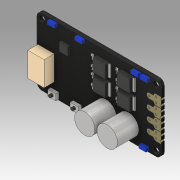
# Autodesk Inventor part: motorcontroller
Saved by Autodesk Inventor 2019.3 (Build 233278000, 278)
## iProperties
Created: 2019-05-13
Part Number: motorcontroller
Material: Generic
Document SubType Name: Modeling
Designer: Dave
Density: 1 g/cm^3
Appearance: Default
Author: Dave
Autodesk Inventor part; units mm, degrees
ref_plane "YZ Plane" through (0, 0, 0) normal (1, 0, 0) x (0, 1, 0)
ref_plane "XZ Plane" through (0, 0, 0) normal (0, 1, 0) x (-1, 0, 0)
ref_plane "XY Plane" through (0, 0, 0) normal (0, 0, 1) x (1, 0, 0)
sketch "Sketch1" plane through (0, 0, 0) normal (0, 0, 1) x (1, 0, 0)
  line L0 (2.5, 0) -> (58.5, 0)
  line L1 (61, 2.5) -> (61, 30.5)
  line L2 (58.5, 33) -> (2.5, 33)
  line L3 (0, 30.5) -> (0, 2.5)
  arc A0 (2.5, 33) -> (0, 30.5) centre (2.5, 30.5) ccw
  arc A1 (61, 30.5) -> (58.5, 33) centre (58.5, 30.5) ccw
  arc A2 (58.5, 0) -> (61, 2.5) centre (58.5, 2.5) ccw
  arc A3 (0, 2.5) -> (2.5, 0) centre (2.5, 2.5) ccw
  circle A4 centre (2.5, 30.5) radius 1.5
  circle A5 centre (2.5, 2.5) radius 1.5
  circle A6 centre (58.5, 30.5) radius 1.5
  circle A7 centre (58.5, 2.5) radius 1.5
  point P0 (0, 0)
  point P1 (61, 33)
  point P2 (61, 0)
  point P3 (0, 33)
  dimension "d0" = 61
  dimension "d1" = 33
  dimension "d2" = 2.5
  dimension "d3" = 3
  dimension "d4" = 56
  dimension "d5" = 28
  constraints: 8 centre point, 8 end point, 8 point on circle, 8 point on line, 8 tangent, 6 equal radius, 4 coincident, 2 parallel, 1 horizontal, 1 perpendicular
  measures "d0" distance of point (61, 33) point (0, 33)
  measures "d1" distance of point (61, 0) point (61, 33)
  measures "d2" radius of A0
  measures "d3" diameter of A4
  measures "d4" distance of A2.centre A3.centre
  measures "d5" distance of A2.centre A1.centre
extrude "Extrusion1" add sketch "Sketch1" along normal blind 1.6
sketch "Sketch2" plane through (0, 0, 1.6) normal (0, 0, 1) x (1, 0, 0)
  circle A0 centre (34, 7) radius 5
  circle A1 centre (45, 7) radius 5
  circle A2 centre (58.5, 2.5) radius 1.5 projected
  circle A3 centre (58.5, 30.5) radius 1.5 projected
  circle A4 centre (2.5, 2.5) radius 1.5 projected
  circle A5 centre (2.5, 30.5) radius 1.5 projected
  line L0 (58.5, 33) -> (2.5, 33) projected
  arc A6 (2.5, 33) -> (0, 30.5) centre (2.5, 30.5) ccw projected
  line L1 (0, 30.5) -> (0, 2.5) projected
  arc A7 (0, 2.5) -> (2.5, 0) centre (2.5, 2.5) ccw projected
  line L2 (2.5, 0) -> (58.5, 0) projected
  arc A8 (58.5, 0) -> (61, 2.5) centre (58.5, 2.5) ccw projected
  line L3 (61, 2.5) -> (61, 30.5) projected
  arc A9 (61, 30.5) -> (58.5, 33) centre (58.5, 30.5) ccw projected
  point P0 (0, 0)
  dimension "d8" = 10
  dimension "d9" = 21
  dimension "d10" = 21
  dimension "d11" = 11
  constraints: 2 centre point, 1 equal radius, 1 horizontal alignment
  measures "d8" diameter of A0
  measures "d10" distance edge to line of A1 L0
  measures "d11" distance edge to line of A1 L3
extrude "Extrusion2" add sketch "Sketch2" along normal blind 10.5 contours A0 | A1
sketch "Sketch3" plane through (0, 0, 1.6) normal (0, 0, 1) x (1, 0, 0)
  line L0 (29.5, 28.5) -> (35.5, 28.5)
  line L1 (35.5, 28.5) -> (35.5, 22.5)
  line L2 (35.5, 22.5) -> (29.5, 22.5)
  line L3 (29.5, 22.5) -> (29.5, 28.5)
  line L4 (29.5, 20.5) -> (35.5, 20.5)
  line L5 (35.5, 20.5) -> (35.5, 14.5)
  line L6 (35.5, 14.5) -> (29.5, 14.5)
  line L7 (29.5, 14.5) -> (29.5, 20.5)
  line L8 (41.5, 28.5) -> (47.5, 28.5)
  line L9 (47.5, 28.5) -> (47.5, 22.5)
  line L10 (47.5, 22.5) -> (41.5, 22.5)
  line L11 (41.5, 22.5) -> (41.5, 28.5)
  line L12 (41.5, 20.5) -> (47.5, 20.5)
  line L13 (47.5, 20.5) -> (47.5, 14.5)
  line L14 (47.5, 14.5) -> (41.5, 14.5)
  line L15 (41.5, 14.5) -> (41.5, 20.5)
  circle A0 centre (34, 7) radius 5 projected
  circle A1 centre (45, 7) radius 5 projected
  circle A2 centre (58.5, 2.5) radius 1.5 projected
  circle A3 centre (58.5, 30.5) radius 1.5 projected
  circle A4 centre (2.5, 2.5) radius 1.5 projected
  circle A5 centre (2.5, 30.5) radius 1.5 projected
  line L16 (58.5, 33) -> (2.5, 33) projected
  arc A6 (2.5, 33) -> (0, 30.5) centre (2.5, 30.5) ccw projected
  line L17 (0, 30.5) -> (0, 2.5) projected
  arc A7 (0, 2.5) -> (2.5, 0) centre (2.5, 2.5) ccw projected
  line L18 (2.5, 0) -> (58.5, 0) projected
  arc A8 (58.5, 0) -> (61, 2.5) centre (58.5, 2.5) ccw projected
  line L19 (61, 2.5) -> (61, 30.5) projected
  arc A9 (61, 30.5) -> (58.5, 33) centre (58.5, 30.5) ccw projected
  point P0 (0, 0)
  dimension "d14" = 6
  dimension "d15" = 6
  dimension "d16" = 2
  dimension "d17" = 4.5
  dimension "d18" = 13.5
  constraints: 32 end point, 8 parallel, 8 point on line, 4 horizontal, 4 perpendicular, 3 equal length, 2 horizontal alignment, 2 vertical alignment
  measures "d14" distance of L2.end L0.start
  measures "d15" distance between parallel lines of L11 L1
  measures "d16" distance between parallel lines of L4 L2
  measures "d17" distance between parallel lines of L16 L0
  measures "d18" distance between parallel lines of L19 L9
extrude "Extrusion3" add sketch "Sketch3" along normal blind 2.1 contours L0 L1 L2 L3 | L4 L5 L6 L7 | L8 L9 L10 L11 | L12 L13 L14 L15
sketch "Sketch4" plane through (0, 0, 1.6) normal (0, 0, 1) x (1, 0, 0)
  line L0 (35.5, 28.5) -> (29.5, 28.5) projected
  line L1 (29.5, 28.5) -> (29.5, 22.5) projected
  line L2 (29.5, 22.5) -> (35.5, 22.5) projected
  line L3 (35.5, 22.5) -> (35.5, 28.5) projected
  line L4 (47.5, 28.5) -> (47.5, 22.5) projected
  line L5 (47.5, 22.5) -> (41.5, 22.5) projected
  line L6 (41.5, 22.5) -> (41.5, 28.5) projected
  line L7 (41.5, 28.5) -> (47.5, 28.5) projected
  line L8 (35.5, 28.5) -> (35.5, 22.5) projected
  line L9 (35.5, 22.5) -> (29.5, 22.5) projected
  line L10 (29.5, 22.5) -> (29.5, 28.5) projected
  line L11 (29.5, 28.5) -> (35.5, 28.5) projected
  line L12 (35.5, 20.5) -> (35.5, 14.5) projected
  line L13 (35.5, 14.5) -> (29.5, 14.5) projected
  line L14 (29.5, 14.5) -> (29.5, 20.5) projected
  line L15 (29.5, 20.5) -> (35.5, 20.5) projected
  line L16 (47.5, 20.5) -> (47.5, 14.5) projected
  line L17 (47.5, 14.5) -> (41.5, 14.5) projected
  line L18 (41.5, 14.5) -> (41.5, 20.5) projected
  line L19 (41.5, 20.5) -> (47.5, 20.5) projected
  circle A0 centre (34, 7) radius 5 projected
  circle A1 centre (45, 7) radius 5 projected
  circle A2 centre (58.5, 2.5) radius 1.5 projected
  circle A3 centre (58.5, 30.5) radius 1.5 projected
  circle A4 centre (2.5, 2.5) radius 1.5 projected
  circle A5 centre (2.5, 30.5) radius 1.5 projected
  line L20 (58.5, 33) -> (2.5, 33) projected
  arc A6 (2.5, 33) -> (0, 30.5) centre (2.5, 30.5) ccw projected
  line L21 (0, 30.5) -> (0, 2.5) projected
  arc A7 (0, 2.5) -> (2.5, 0) centre (2.5, 2.5) ccw projected
  line L22 (2.5, 0) -> (58.5, 0) projected
  arc A8 (58.5, 0) -> (61, 2.5) centre (58.5, 2.5) ccw projected
  line L23 (61, 2.5) -> (61, 30.5) projected
  arc A9 (61, 30.5) -> (58.5, 33) centre (58.5, 30.5) ccw projected
  line L24 (35.5, 20.5) -> (29.5, 20.5) projected
  line L25 (29.5, 20.5) -> (29.5, 14.5) projected
  line L26 (29.5, 14.5) -> (35.5, 14.5) projected
  line L27 (35.5, 14.5) -> (35.5, 20.5) projected
  line L28 (47.5, 20.5) -> (41.5, 20.5) projected
  line L29 (41.5, 20.5) -> (41.5, 14.5) projected
  line L30 (41.5, 14.5) -> (47.5, 14.5) projected
  line L31 (47.5, 14.5) -> (47.5, 20.5) projected
  line L32 (47.5, 28.5) -> (41.5, 28.5) projected
  line L33 (41.5, 28.5) -> (41.5, 22.5) projected
  line L34 (41.5, 22.5) -> (47.5, 22.5) projected
  line L35 (47.5, 22.5) -> (47.5, 28.5) projected
  line L36 (35.5, 28.5) -> (36.5, 28.5)
  line L37 (36.5, 28.5) -> (36.5, 22.5)
  line L38 (36.5, 22.5) -> (35.5, 22.5)
  line L39 (35.5, 22.5) -> (35.5, 28.5)
  line L40 (35.5, 20.5) -> (36.5, 20.5)
  line L41 (36.5, 20.5) -> (36.5, 14.5)
  line L42 (36.5, 14.5) -> (35.5, 14.5)
  line L43 (35.5, 14.5) -> (35.5, 20.5)
  line L44 (47.5, 28.5) -> (48.5, 28.5)
  line L45 (48.5, 28.5) -> (48.5, 22.5)
  line L46 (48.5, 22.5) -> (47.5, 22.5)
  line L47 (47.5, 22.5) -> (47.5, 28.5)
  line L48 (47.5, 20.5) -> (48.5, 20.5)
  line L49 (48.5, 20.5) -> (48.5, 14.5)
  line L50 (48.5, 14.5) -> (47.5, 14.5)
  line L51 (47.5, 14.5) -> (47.5, 20.5)
  line L52 (29.5, 22.5) -> (35.5, 22.5) projected
  point P0 (0, 0)
  dimension "d21" = 1
  constraints: 32 end point, 8 parallel, 4 horizontal, 4 perpendicular, 4 point on line, 2 equal length, 1 collinear
  measures "d21" distance of L8.start L36.end
extrude "Extrusion4" add sketch "Sketch4" along normal blind 0.6 contours L3 L2 L1 L0 | L36 L37 L38 L3 | L44 L45 L46 L4 | L40 L41 L42 L12 | L48 L49 L50 L16
sketch "Sketch5" plane through (0, 0, 1.6) normal (0, 0, 1) x (1, 0, 0)
  line L0 (35.5, 28.5) -> (29.5, 28.5) projected
  line L1 (29.5, 28.5) -> (29.5, 22.5) projected
  line L2 (29.5, 22.5) -> (35.5, 22.5) projected
  line L3 (35.5, 22.5) -> (35.5, 28.5) projected
  line L4 (35.5, 20.5) -> (29.5, 20.5) projected
  line L5 (29.5, 20.5) -> (29.5, 14.5) projected
  line L6 (29.5, 14.5) -> (35.5, 14.5) projected
  line L7 (35.5, 14.5) -> (35.5, 20.5) projected
  line L8 (47.5, 20.5) -> (41.5, 20.5) projected
  line L9 (41.5, 20.5) -> (41.5, 14.5) projected
  line L10 (41.5, 14.5) -> (47.5, 14.5) projected
  line L11 (47.5, 14.5) -> (47.5, 20.5) projected
  line L12 (47.5, 28.5) -> (41.5, 28.5) projected
  line L13 (41.5, 28.5) -> (41.5, 22.5) projected
  line L14 (41.5, 22.5) -> (47.5, 22.5) projected
  line L15 (47.5, 22.5) -> (47.5, 28.5) projected
  line L16 (29.5, 28.25) -> (27, 28.25)
  line L17 (27, 28.25) -> (27, 27.25)
  line L18 (27, 27.25) -> (29.5, 27.25)
  line L19 (29.5, 27.25) -> (29.5, 28.25)
  line L20 (29.5, 23.75) -> (27, 23.75)
  line L21 (27, 23.75) -> (27, 22.75)
  line L22 (27, 22.75) -> (29.5, 22.75)
  line L23 (29.5, 22.75) -> (29.5, 23.75)
  line L24 (29.5, 20.25) -> (27, 20.25)
  line L25 (27, 20.25) -> (27, 19.25)
  line L26 (27, 19.25) -> (29.5, 19.25)
  line L27 (29.5, 19.25) -> (29.5, 20.25)
  line L28 (29.5, 15.75) -> (27, 15.75)
  line L29 (27, 15.75) -> (27, 14.75)
  line L30 (27, 14.75) -> (29.5, 14.75)
  line L31 (29.5, 14.75) -> (29.5, 15.75)
  line L32 (41.5, 28.25) -> (39, 28.25)
  line L33 (39, 28.25) -> (39, 27.25)
  line L34 (39, 27.25) -> (41.5, 27.25)
  line L35 (41.5, 27.25) -> (41.5, 28.25)
  line L36 (41.5, 23.75) -> (39, 23.75)
  line L37 (39, 23.75) -> (39, 22.75)
  line L38 (39, 22.75) -> (41.5, 22.75)
  line L39 (41.5, 22.75) -> (41.5, 23.75)
  line L40 (41.5, 20.25) -> (39, 20.25)
  line L41 (39, 20.25) -> (39, 19.25)
  line L42 (39, 19.25) -> (41.5, 19.25)
  line L43 (41.5, 19.25) -> (41.5, 20.25)
  line L44 (41.5, 15.75) -> (39, 15.75)
  line L45 (39, 15.75) -> (39, 14.75)
  line L46 (39, 14.75) -> (41.5, 14.75)
  line L47 (41.5, 14.75) -> (41.5, 15.75)
  point P0 (0, 0)
  dimension "d24" = 1
  dimension "d25" = 2.5
  dimension "d26" = 3.5
  dimension "d27" = 3.5
  dimension "d28" = 6
  dimension "d29" = 5.5
  dimension "d30" = 0.25
  dimension "d31" = 0.25
  constraints: 64 end point, 21 point on line, 16 parallel, 8 horizontal, 8 perpendicular, 4 equal length, 1 collinear
  measures "d24" distance between parallel lines of L18 L16
  measures "d25" distance of L16.start L16.end
  measures "d26" distance between parallel lines of L36 L34
  measures "d27" distance between parallel lines of L44 L42
  measures "d28" distance of L12.end L13.end
  measures "d29" distance between parallel lines of L38 L32
  measures "d30" distance between parallel lines of L12 L32
  measures "d31" distance between parallel lines of L4 L24
extrude "Extrusion5" add sketch "Sketch5" along normal blind 1.7 contours L1 L18 L17 L16 | L22 L21 L20 L1 | L5 L26 L25 L24 | L30 L29 L28 L5 | L9 L42 L41 L40 | L46 L45 L44 L9 | L13 L34 L33 L32 | L38 L37 L36 L13
sketch "Sketch6" plane through (39, 28.25, 1.6) normal (0, 1, 0) x (1, 0, 0)
  line L0 (2.5, 0) -> (9.5, 0) projected
  line L1 (2.5, 0) -> (2.5, -2.1) projected
  line L2 (8.5, -2.1) -> (2.5, -2.1) projected
  line L3 (8.5, -0.6) -> (8.5, -2.1) projected
  line L4 (9.5, -0.6) -> (8.5, -0.6) projected
  line L5 (9.5, 0) -> (9.5, -0.6) projected
  line L6 (-9.5, 0) -> (-9.5, -2.1) projected
  line L7 (-3.5, -2.1) -> (-9.5, -2.1) projected
  line L8 (-3.5, -0.6) -> (-3.5, -2.1) projected
  line L9 (-2.5, -0.6) -> (-3.5, -0.6) projected
  line L10 (-2.5, 0) -> (-2.5, -0.6) projected
  line L11 (-9.5, 0) -> (-2.5, 0) projected
  line L12 (-12, 0) -> (-9.5, 0) projected
  line L13 (-12, 0) -> (-12, -1.7) projected
  line L14 (-9.5, -1.7) -> (-12, -1.7) projected
  line L15 (-9.5, 0) -> (-9.5, -1.7) projected
  line L16 (0, 0) -> (2.5, 0) projected
  line L17 (0, 0) -> (0, -1.7) projected
  line L18 (2.5, -1.7) -> (0, -1.7) projected
  line L19 (2.5, 0) -> (2.5, -1.7) projected
  line L20 (2.5, -1.7) -> (1.7, -1.7)
  line L21 (1.7, -1.7) -> (0.8, -0.5)
  line L22 (0.8, -0.5) -> (0, -0.5)
  line L23 (2.5, -1.2) -> (1.95, -1.2)
  line L24 (1.95, -1.2) -> (1.05, 0)
  line L25 (0, -0.5) -> (0, 0)
  line L26 (1.05, 0) -> (0, 0)
  line L27 (2.5, -1.7) -> (2.5, -1.2)
  line L28 (1.7, -1.7) -> (0, -1.7)
  line L29 (0, -1.7) -> (0, -0.5)
  line L30 (2.5, -1.2) -> (2.5, 0)
  line L31 (2.5, 0) -> (1.05, 0)
  line L32 (-9.5, -1.7) -> (-10.3, -1.7)
  line L33 (-10.3, -1.7) -> (-11.2, -0.5)
  line L34 (-11.2, -0.5) -> (-12, -0.5)
  line L35 (-9.5, -1.2) -> (-10.05, -1.2)
  line L36 (-10.05, -1.2) -> (-10.95, 0)
  line L37 (-10.95, 0) -> (-12, 0)
  line L38 (-12, 0) -> (-12, -0.5)
  line L39 (-9.5, -1.2) -> (-9.5, 0)
  line L40 (-9.5, 0.0258) -> (-10.95, 0)
  line L41 (-10.3, -1.7) -> (-12, -1.7)
  line L42 (-12, -1.7) -> (-12, -0.5)
  point P0 (-39, 1.6)
  dimension "d34" = 0.5
  dimension "d35" = 0.5
  dimension "d36" = 0.5
  dimension "d37" = 0.8
  dimension "d39" = 0.8
  dimension "d42" = 0.5
  dimension "d43" = 0.5
  dimension "d44" = 0.5
  dimension "d45" = 0.8
  dimension "d46" = 0.8
  constraints: 46 end point, 9 point on line, 7 collinear, 7 perpendicular, 2 horizontal, 2 parallel
  measures "d34" distance between parallel lines of L24 L21
  measures "d35" distance between parallel lines of L23 L20
  measures "d36" distance between parallel lines of L16 L22
  measures "d37" distance of L18.start L20.end
  measures "d39" distance of L21.end L22.end
  measures "d42" distance between parallel lines of L32 L35
  measures "d43" distance between parallel lines of L12 L34
  measures "d44" distance between parallel lines of L33 L36
  measures "d45" distance of L14.start L32.end
  measures "d46" distance of L33.end L34.end
extrude "Extrusion6" cut sketch "Sketch6" against normal up to surface (13.5 mm away) contours L1 L23 L24 L16 | L18 L17 L22 L21 | L6 L35 L36 L12 | L14 L13 L34 L33
sketch "Sketch7" plane through (0, 0, 1.6) normal (0, 0, 1) x (1, 0, 0)
  line L0 (6.5, 32.5) -> (10, 32.5)
  line L1 (10, 32.5) -> (10, 31)
  line L2 (10, 31) -> (6.5, 31)
  line L3 (6.5, 31) -> (6.5, 32.5)
  line L4 (20, 32.5) -> (23.5, 32.5)
  line L5 (23.5, 32.5) -> (23.5, 31)
  line L6 (23.5, 31) -> (20, 31)
  line L7 (20, 31) -> (20, 32.5)
  line L8 (51.5, 2.2778) -> (55, 2.2778)
  line L9 (55, 2.2778) -> (55, 0.7778)
  line L10 (55, 0.7778) -> (51.5, 0.7778)
  line L11 (51.5, 0.7778) -> (51.5, 2.2778)
  line L12 (58.5, 33) -> (2.5, 33) projected
  line L13 (0, 30.5) -> (0, 2.5) projected
  line L14 (61, 2.5) -> (61, 30.5) projected
  line L15 (2.5, 0) -> (58.5, 0) projected
  line L16 (47.5, 32) -> (51, 32)
  line L17 (51, 32) -> (51, 30.5)
  line L18 (51, 30.5) -> (47.5, 30.5)
  line L19 (47.5, 30.5) -> (47.5, 32)
  line L20 (52, 32) -> (55.5, 32)
  line L21 (55.5, 32) -> (55.5, 30.5)
  line L22 (55.5, 30.5) -> (52, 30.5)
  line L23 (52, 30.5) -> (52, 32)
  point P0 (0, 0)
  dimension "d47" = 3.5
  dimension "d48" = 1.5
  dimension "d49" = 10
  dimension "d52" = 6.5
  dimension "d54" = 6
  dimension "d55" = 0.7778
  dimension "d56" = 0.5
  dimension "d57" = 1
  dimension "d58" = 5.5
  dimension "d59" = 1
  constraints: 40 end point, 10 parallel, 6 equal length, 5 horizontal, 5 perpendicular, 4 point on line
  measures "d47" distance of L1.end L2.end
  measures "d48" distance of L2.end L0.start
  measures "d49" distance between parallel lines of L7 L1
  measures "d52" distance between parallel lines of L13 L3
  measures "d54" distance between parallel lines of L14 L9
  measures "d55" distance between parallel lines of L15 L10
  measures "d56" distance between parallel lines of L12 L0
  measures "d57" distance between parallel lines of L12 L16
  measures "d58" distance between parallel lines of L14 L21
  measures "d59" distance between parallel lines of L23 L17
extrude "Extrusion7" add sketch "Sketch7" along normal blind 1.5
sketch "Sketch8" plane through (0, 0, 1.6) normal (0, 0, 1) x (1, 0, 0)
  line L0 (0.5, 18.7) -> (8.5, 18.7)
  line L1 (8.5, 18.7) -> (8.5, 6.7)
  line L2 (8.5, 6.7) -> (0.5, 6.7)
  line L3 (0.5, 6.7) -> (0.5, 18.7)
  line L4 (0, 30.5) -> (0, 2.5) projected
  line L5 (58.5, 33) -> (2.5, 33) projected
  point P0 (0, 0)
  dimension "d62" = 12
  dimension "d63" = 8
  dimension "d64" = 0.5
  dimension "d65" = 14.3
  constraints: 8 end point, 2 parallel, 1 horizontal, 1 perpendicular
  measures "d62" distance of L0.end L1.end
  measures "d63" distance of L0.start L0.end
  measures "d64" distance between parallel lines of L4 L3
  measures "d65" distance between parallel lines of L5 L0
extrude "Extrusion8" add sketch "Sketch8" along normal blind 5
sketch "Sketch9" plane through (0, 0, 1.6) normal (0, 0, 1) x (1, 0, 0)
  line L0 (6.8, 3.5) -> (10.8, 3.5)
  line L1 (10.8, 3.5) -> (10.8, 0.5)
  line L2 (10.8, 0.5) -> (6.8, 0.5)
  line L3 (6.8, 0.5) -> (6.8, 3.5)
  line L4 (17.8, 3.5) -> (21.8, 3.5)
  line L5 (21.8, 3.5) -> (21.8, 0.5)
  line L6 (21.8, 0.5) -> (17.8, 0.5)
  line L7 (17.8, 0.5) -> (17.8, 3.5)
  line L8 (0, 30.5) -> (0, 2.5) projected
  line L9 (2.5, 0) -> (58.5, 0) projected
  point P0 (0, 0)
  dimension "d68" = 4
  dimension "d69" = 4
  dimension "d70" = 3
  dimension "d71" = 7
  dimension "d72" = 6.8
  dimension "d73" = 0.5
  constraints: 16 end point, 4 parallel, 2 horizontal, 2 perpendicular, 2 point on line
  measures "d68" distance of L0.start L0.end
  measures "d69" distance of L4.start L4.end
  measures "d70" distance of L0.end L1.end
  measures "d71" distance between parallel lines of L7 L1
  measures "d72" distance between parallel lines of L8 L3
  measures "d73" distance between parallel lines of L9 L6
extrude "Extrusion9" add sketch "Sketch9" along normal blind 1.5
sketch "Sketch10" plane through (0, 0, 3.1) normal (0, 0, 1) x (1, 0, 0)
  line L0 (10.8, 3.5) -> (6.8, 3.5) projected
  line L1 (6.8, 3.5) -> (6.8, 0.5) projected
  line L2 (6.8, 0.5) -> (10.8, 0.5) projected
  line L3 (10.8, 0.5) -> (10.8, 3.5) projected
  line L4 (21.8, 3.5) -> (17.8, 3.5) projected
  line L5 (17.8, 3.5) -> (17.8, 0.5) projected
  line L6 (17.8, 0.5) -> (21.8, 0.5) projected
  line L7 (21.8, 0.5) -> (21.8, 3.5) projected
  circle A0 centre (8.8, 2) radius 0.75
  circle A1 centre (19.8, 2) radius 0.75
  point P0 (0, 0)
  point P1 (10.8, 2)
  point P2 (21.8, 2)
  point P3 (8.8, 3.5)
  point P4 (19.8, 3.5)
  dimension "d76" = 1.5
  constraints: 4 midpoint, 2 centre point, 2 horizontal alignment, 2 vertical alignment, 1 equal radius
  measures "d76" diameter of A0
extrude "Extrusion10" add sketch "Sketch10" along normal blind 1 contours A0 | A1
sketch "Sketch11" plane through (0, 0, 1.6) normal (0, 0, 1) x (1, 0, 0)
  line L0 (12, 26) -> (16, 26)
  line L1 (16, 26) -> (16, 22)
  line L2 (16, 22) -> (12, 22)
  line L3 (12, 22) -> (12, 26)
  line L4 (58.5, 33) -> (2.5, 33) projected
  line L5 (0, 30.5) -> (0, 2.5) projected
  point P0 (0, 0)
  dimension "d79" = 4
  dimension "d80" = 4
  dimension "d81" = 7
  dimension "d82" = 12
  constraints: 8 end point, 2 parallel, 1 horizontal, 1 perpendicular
  measures "d79" distance of L0.start L0.end
  measures "d80" distance of L0.end L1.end
  measures "d81" distance between parallel lines of L4 L0
  measures "d82" distance between parallel lines of L5 L3
extrude "Extrusion11" add sketch "Sketch11" along normal blind 1
sketch "Sketch12" plane through (0, 0, 1.6) normal (0, 0, 1) x (1, 0, 0)
  circle A0 centre (58.46, 25.39) radius 0.4
  line L0 (16, 26) -> (16, 22) projected
  line L1 (16, 22) -> (12, 22) projected
  line L2 (12, 22) -> (12, 26) projected
  line L3 (12, 26) -> (16, 26) projected
  line L4 (10.8, 3.5) -> (10.8, 0.5) projected
  line L5 (10.8, 0.5) -> (6.8, 0.5) projected
  line L6 (6.8, 0.5) -> (6.8, 3.5) projected
  line L7 (6.8, 3.5) -> (10.8, 3.5) projected
  line L8 (21.8, 3.5) -> (21.8, 0.5) projected
  line L9 (21.8, 0.5) -> (17.8, 0.5) projected
  line L10 (17.8, 0.5) -> (17.8, 3.5) projected
  line L11 (17.8, 3.5) -> (21.8, 3.5) projected
  line L12 (8.5, 18.7) -> (8.5, 6.7) projected
  line L13 (8.5, 6.7) -> (0.5, 6.7) projected
  line L14 (0.5, 6.7) -> (0.5, 18.7) projected
  line L15 (0.5, 18.7) -> (8.5, 18.7) projected
  line L16 (51, 32) -> (51, 30.5) projected
  line L17 (51, 30.5) -> (47.5, 30.5) projected
  line L18 (47.5, 30.5) -> (47.5, 32) projected
  line L19 (47.5, 32) -> (51, 32) projected
  line L20 (23.5, 32.5) -> (23.5, 31) projected
  line L21 (23.5, 31) -> (20, 31) projected
  line L22 (20, 31) -> (20, 32.5) projected
  line L23 (20, 32.5) -> (23.5, 32.5) projected
  line L24 (10, 32.5) -> (10, 31) projected
  line L25 (10, 31) -> (6.5, 31) projected
  line L26 (6.5, 31) -> (6.5, 32.5) projected
  line L27 (6.5, 32.5) -> (10, 32.5) projected
  line L28 (55, 2.2778) -> (55, 0.7778) projected
  line L29 (55, 0.7778) -> (51.5, 0.7778) projected
  line L30 (51.5, 0.7778) -> (51.5, 2.2778) projected
  line L31 (51.5, 2.2778) -> (55, 2.2778) projected
  line L32 (55.5, 32) -> (55.5, 30.5) projected
  line L33 (55.5, 30.5) -> (52, 30.5) projected
  line L34 (52, 30.5) -> (52, 32) projected
  line L35 (52, 32) -> (55.5, 32) projected
  line L36 (28.05, 14.75) -> (27, 14.75) projected
  line L37 (27, 14.75) -> (27, 15.75) projected
  line L38 (27, 15.75) -> (28.05, 15.75) projected
  line L39 (28.05, 15.75) -> (28.05, 14.75) projected
  line L40 (29.5, 22.5) -> (29.5, 28.5) projected
  line L41 (29.5, 28.5) -> (36.5, 28.5) projected
  line L42 (36.5, 28.5) -> (36.5, 22.5) projected
  line L43 (36.5, 22.5) -> (29.5, 22.5) projected
  line L44 (28.05, 27.25) -> (27, 27.25) projected
  line L45 (27, 27.25) -> (27, 28.25) projected
  line L46 (27, 28.25) -> (28.05, 28.25) projected
  line L47 (28.05, 28.25) -> (28.05, 27.25) projected
  line L48 (28.05, 19.25) -> (27, 19.25) projected
  line L49 (27, 19.25) -> (27, 20.25) projected
  line L50 (27, 20.25) -> (28.05, 20.25) projected
  line L51 (28.05, 20.25) -> (28.05, 19.25) projected
  line L52 (40.05, 14.75) -> (39, 14.75) projected
  line L53 (39, 14.75) -> (39, 15.75) projected
  line L54 (39, 15.75) -> (40.05, 15.75) projected
  line L55 (40.05, 15.75) -> (40.05, 14.75) projected
  line L56 (41.5, 22.5) -> (41.5, 28.5) projected
  line L57 (41.5, 28.5) -> (48.5, 28.5) projected
  line L58 (48.5, 28.5) -> (48.5, 22.5) projected
  line L59 (48.5, 22.5) -> (41.5, 22.5) projected
  line L60 (40.05, 19.25) -> (39, 19.25) projected
  line L61 (39, 19.25) -> (39, 20.25) projected
  line L62 (39, 20.25) -> (40.05, 20.25) projected
  line L63 (40.05, 20.25) -> (40.05, 19.25) projected
  line L64 (40.05, 22.75) -> (39, 22.75) projected
  line L65 (39, 22.75) -> (39, 23.75) projected
  line L66 (39, 23.75) -> (40.05, 23.75) projected
  line L67 (40.05, 23.75) -> (40.05, 22.75) projected
  line L68 (28.05, 23.75) -> (28.05, 22.75) projected
  line L69 (28.05, 22.75) -> (27, 22.75) projected
  line L70 (27, 22.75) -> (27, 23.75) projected
  line L71 (27, 23.75) -> (28.05, 23.75) projected
  line L72 (41.5, 14.5) -> (41.5, 20.5) projected
  line L73 (41.5, 20.5) -> (48.5, 20.5) projected
  line L74 (48.5, 20.5) -> (48.5, 14.5) projected
  line L75 (48.5, 14.5) -> (41.5, 14.5) projected
  line L76 (29.5, 14.5) -> (29.5, 20.5) projected
  line L77 (29.5, 20.5) -> (36.5, 20.5) projected
  line L78 (36.5, 20.5) -> (36.5, 14.5) projected
  line L79 (36.5, 14.5) -> (29.5, 14.5) projected
  line L80 (40.05, 28.25) -> (40.05, 27.25) projected
  line L81 (40.05, 27.25) -> (39, 27.25) projected
  line L82 (39, 27.25) -> (39, 28.25) projected
  line L83 (39, 28.25) -> (40.05, 28.25) projected
  circle A1 centre (34, 7) radius 5 projected
  circle A2 centre (45, 7) radius 5 projected
  circle A3 centre (58.5, 2.5) radius 1.5 projected
  circle A4 centre (58.5, 30.5) radius 1.5 projected
  circle A5 centre (2.5, 2.5) radius 1.5 projected
  circle A6 centre (2.5, 30.5) radius 1.5 projected
  line L84 (58.5, 33) -> (2.5, 33) projected
  arc A7 (2.5, 33) -> (0, 30.5) centre (2.5, 30.5) ccw projected
  line L85 (0, 30.5) -> (0, 2.5) projected
  arc A8 (0, 2.5) -> (2.5, 0) centre (2.5, 2.5) ccw projected
  line L86 (2.5, 0) -> (58.5, 0) projected
  arc A9 (58.5, 0) -> (61, 2.5) centre (58.5, 2.5) ccw projected
  line L87 (61, 2.5) -> (61, 30.5) projected
  arc A10 (61, 30.5) -> (58.5, 33) centre (58.5, 30.5) ccw projected
  circle A11 centre (58.46, 22.85) radius 0.4
  circle A12 centre (58.46, 20.31) radius 0.4
  circle A13 centre (58.46, 17.77) radius 0.4
  circle A14 centre (58.46, 15.23) radius 0.4
  circle A15 centre (58.46, 12.69) radius 0.4
  circle A16 centre (58.46, 10.15) radius 0.4
  circle A17 centre (58.46, 7.61) radius 0.4
  circle A18 centre (61, 25.39) radius 0.4
  circle A19 centre (61, 22.85) radius 0.4
  circle A20 centre (61, 20.31) radius 0.4
  circle A21 centre (61, 17.77) radius 0.4
  circle A22 centre (61, 15.23) radius 0.4
  circle A23 centre (61, 12.69) radius 0.4
  circle A24 centre (61, 10.15) radius 0.4
  circle A25 centre (61, 7.61) radius 0.4
  circle A26 centre (55.16, 24.12) radius 0.4
  circle A27 centre (55.16, 19.04) radius 0.4
  circle A28 centre (55.16, 13.96) radius 0.4
  circle A29 centre (55.16, 8.88) radius 0.4
  point P0 (0, 0)
  dimension "d85" = 0.8
  dimension "d88" = 2.54
  dimension "d91" = 2.54
  dimension "d94" = 7.61
  dimension "d95" = 7.61
  dimension "d98" = 5.08
  dimension "d103" = 1.27
  dimension "d104" = 3.3
  constraints: 20 centre point, 2 vertical, 1 equal radius, 1 horizontal, 1 point on line, 36 other
  measures "d85" diameter of A0
  measures "d88" distance of A0.centre A11.centre
  measures "d91" distance of A0.centre A18.centre
  measures "d94" distance from line of L86 A17.centre
  measures "d95" distance from line of L84 A0.centre
  measures "d98" distance of A26.centre A27.centre
  measures "d103" vertical distance of A0.centre A26.centre
  measures "d104" horizontal distance of A0.centre A26.centre
extrude "Extrusion12" cut sketch "Sketch12" against normal through all contours A0 | A18 L87 | L87 A18 | A19 L87 | L87 A19 | A20 L87 | L87 A20 | A25 L87 | L87 A25 | A21 L87 | L87 A21 | A24 L87 | L87 A24 | A22 L87 | L87 A22 | A23 L87 | L87 A23 | A11 | A12 | A13 | A14 | A15 | A16 | A17 | A26 | A27 | A28 | A29
sketch "Sketch13" plane through (0, 0, 1.6) normal (0, 0, 1) x (1, 0, 0)
  arc A0 (61, 8.01) -> (61, 7.21) centre (61, 7.61) ccw projected
  line L0 (61, 8.01) -> (61, 9.75) projected
  arc A1 (61, 10.55) -> (61, 9.75) centre (61, 10.15) ccw projected
  line L1 (61, 10.55) -> (61, 12.29) projected
  arc A2 (61, 13.09) -> (61, 12.29) centre (61, 12.69) ccw projected
  line L2 (61, 13.09) -> (61, 14.83) projected
  arc A3 (61, 15.63) -> (61, 14.83) centre (61, 15.23) ccw projected
  line L3 (61, 15.63) -> (61, 17.37) projected
  arc A4 (61, 18.17) -> (61, 17.37) centre (61, 17.77) ccw projected
  line L4 (61, 18.17) -> (61, 19.91) projected
  arc A5 (61, 20.71) -> (61, 19.91) centre (61, 20.31) ccw projected
  line L5 (61, 20.71) -> (61, 22.45) projected
  arc A6 (61, 23.25) -> (61, 22.45) centre (61, 22.85) ccw projected
  line L6 (61, 23.25) -> (61, 24.99) projected
  arc A7 (61, 25.79) -> (61, 24.99) centre (61, 25.39) ccw projected
  line L7 (61, 25.79) -> (61, 30.5) projected
  arc A8 (61, 30.5) -> (58.5, 33) centre (58.5, 30.5) ccw projected
  line L8 (58.5, 33) -> (2.5, 33) projected
  arc A9 (2.5, 33) -> (0, 30.5) centre (2.5, 30.5) ccw projected
  line L9 (0, 30.5) -> (0, 2.5) projected
  arc A10 (0, 2.5) -> (2.5, 0) centre (2.5, 2.5) ccw projected
  line L10 (2.5, 0) -> (58.5, 0) projected
  arc A11 (58.5, 0) -> (61, 2.5) centre (58.5, 2.5) ccw projected
  line L11 (61, 2.5) -> (61, 7.21) projected
  circle A12 centre (55.16, 8.88) radius 0.4 projected
  circle A13 centre (55.16, 19.04) radius 0.4 projected
  circle A14 centre (58.46, 7.61) radius 0.4 projected
  circle A15 centre (58.46, 12.69) radius 0.4 projected
  circle A16 centre (58.46, 17.77) radius 0.4 projected
  circle A17 centre (58.46, 22.85) radius 0.4 projected
  circle A18 centre (58.46, 25.39) radius 0.4 projected
  circle A19 centre (58.46, 20.31) radius 0.4 projected
  circle A20 centre (58.46, 15.23) radius 0.4 projected
  circle A21 centre (58.46, 10.15) radius 0.4 projected
  circle A22 centre (55.16, 24.12) radius 0.4 projected
  circle A23 centre (55.16, 13.96) radius 0.4 projected
  line L12 (16, 26) -> (16, 22) projected
  line L13 (16, 22) -> (12, 22) projected
  line L14 (12, 22) -> (12, 26) projected
  line L15 (12, 26) -> (16, 26) projected
  line L16 (10.8, 3.5) -> (10.8, 0.5) projected
  line L17 (10.8, 0.5) -> (6.8, 0.5) projected
  line L18 (6.8, 0.5) -> (6.8, 3.5) projected
  line L19 (6.8, 3.5) -> (10.8, 3.5) projected
  line L20 (21.8, 3.5) -> (21.8, 0.5) projected
  line L21 (21.8, 0.5) -> (17.8, 0.5) projected
  line L22 (17.8, 0.5) -> (17.8, 3.5) projected
  line L23 (17.8, 3.5) -> (21.8, 3.5) projected
  line L24 (8.5, 18.7) -> (8.5, 6.7) projected
  line L25 (8.5, 6.7) -> (0.5, 6.7) projected
  line L26 (0.5, 6.7) -> (0.5, 18.7) projected
  line L27 (0.5, 18.7) -> (8.5, 18.7) projected
  line L28 (51, 32) -> (51, 30.5) projected
  line L29 (51, 30.5) -> (47.5, 30.5) projected
  line L30 (47.5, 30.5) -> (47.5, 32) projected
  line L31 (47.5, 32) -> (51, 32) projected
  line L32 (23.5, 32.5) -> (23.5, 31) projected
  line L33 (23.5, 31) -> (20, 31) projected
  line L34 (20, 31) -> (20, 32.5) projected
  line L35 (20, 32.5) -> (23.5, 32.5) projected
  line L36 (10, 32.5) -> (10, 31) projected
  line L37 (10, 31) -> (6.5, 31) projected
  line L38 (6.5, 31) -> (6.5, 32.5) projected
  line L39 (6.5, 32.5) -> (10, 32.5) projected
  line L40 (55, 2.2778) -> (55, 0.7778) projected
  line L41 (55, 0.7778) -> (51.5, 0.7778) projected
  line L42 (51.5, 0.7778) -> (51.5, 2.2778) projected
  line L43 (51.5, 2.2778) -> (55, 2.2778) projected
  line L44 (55.5, 32) -> (55.5, 30.5) projected
  line L45 (55.5, 30.5) -> (52, 30.5) projected
  line L46 (52, 30.5) -> (52, 32) projected
  line L47 (52, 32) -> (55.5, 32) projected
  line L48 (28.05, 14.75) -> (27, 14.75) projected
  line L49 (27, 14.75) -> (27, 15.75) projected
  line L50 (27, 15.75) -> (28.05, 15.75) projected
  line L51 (28.05, 15.75) -> (28.05, 14.75) projected
  line L52 (29.5, 22.5) -> (29.5, 28.5) projected
  line L53 (29.5, 28.5) -> (36.5, 28.5) projected
  line L54 (36.5, 28.5) -> (36.5, 22.5) projected
  line L55 (36.5, 22.5) -> (29.5, 22.5) projected
  line L56 (28.05, 27.25) -> (27, 27.25) projected
  line L57 (27, 27.25) -> (27, 28.25) projected
  line L58 (27, 28.25) -> (28.05, 28.25) projected
  line L59 (28.05, 28.25) -> (28.05, 27.25) projected
  line L60 (28.05, 19.25) -> (27, 19.25) projected
  line L61 (27, 19.25) -> (27, 20.25) projected
  line L62 (27, 20.25) -> (28.05, 20.25) projected
  line L63 (28.05, 20.25) -> (28.05, 19.25) projected
  line L64 (40.05, 14.75) -> (39, 14.75) projected
  line L65 (39, 14.75) -> (39, 15.75) projected
  line L66 (39, 15.75) -> (40.05, 15.75) projected
  line L67 (40.05, 15.75) -> (40.05, 14.75) projected
  line L68 (41.5, 22.5) -> (41.5, 28.5) projected
  line L69 (41.5, 28.5) -> (48.5, 28.5) projected
  line L70 (48.5, 28.5) -> (48.5, 22.5) projected
  line L71 (48.5, 22.5) -> (41.5, 22.5) projected
  line L72 (40.05, 19.25) -> (39, 19.25) projected
  line L73 (39, 19.25) -> (39, 20.25) projected
  line L74 (39, 20.25) -> (40.05, 20.25) projected
  line L75 (40.05, 20.25) -> (40.05, 19.25) projected
  line L76 (40.05, 22.75) -> (39, 22.75) projected
  line L77 (39, 22.75) -> (39, 23.75) projected
  line L78 (39, 23.75) -> (40.05, 23.75) projected
  line L79 (40.05, 23.75) -> (40.05, 22.75) projected
  line L80 (28.05, 23.75) -> (28.05, 22.75) projected
  line L81 (28.05, 22.75) -> (27, 22.75) projected
  line L82 (27, 22.75) -> (27, 23.75) projected
  line L83 (27, 23.75) -> (28.05, 23.75) projected
  line L84 (41.5, 14.5) -> (41.5, 20.5) projected
  line L85 (41.5, 20.5) -> (48.5, 20.5) projected
  line L86 (48.5, 20.5) -> (48.5, 14.5) projected
  line L87 (48.5, 14.5) -> (41.5, 14.5) projected
  line L88 (29.5, 14.5) -> (29.5, 20.5) projected
  line L89 (29.5, 20.5) -> (36.5, 20.5) projected
  line L90 (36.5, 20.5) -> (36.5, 14.5) projected
  line L91 (36.5, 14.5) -> (29.5, 14.5) projected
  line L92 (40.05, 28.25) -> (40.05, 27.25) projected
  line L93 (40.05, 27.25) -> (39, 27.25) projected
  line L94 (39, 27.25) -> (39, 28.25) projected
  line L95 (39, 28.25) -> (40.05, 28.25) projected
  circle A24 centre (34, 7) radius 5 projected
  circle A25 centre (45, 7) radius 5 projected
  circle A26 centre (58.5, 2.5) radius 1.5 projected
  circle A27 centre (58.5, 30.5) radius 1.5 projected
  circle A28 centre (2.5, 2.5) radius 1.5 projected
  circle A29 centre (2.5, 30.5) radius 1.5 projected
  line L96 (61, 26.57) -> (58.46, 26.57)
  line L97 (61, 21.67) -> (58.46, 21.67)
  line L98 (61, 20.71) -> (61, 22.45) projected
  arc A30 (58.46, 26.57) -> (57.2802, 25.37) centre (58.46, 25.39) ccw
  arc A31 (57.2802, 22.87) -> (58.46, 21.67) centre (58.46, 22.85) ccw
  arc A32 (55.16, 25.37) -> (55.16, 22.87) centre (55.16, 24.12) ccw
  line L99 (55.16, 25.37) -> (57.2802, 25.37)
  line L100 (55.16, 22.87) -> (57.2802, 22.87)
  line L101 (61, 26.57) -> (61, 21.67)
  line L102 (61, 16.59) -> (58.46, 16.59)
  line L103 (61, 21.49) -> (61, 16.59)
  line L104 (61, 21.49) -> (58.46, 21.49)
  arc A33 (58.46, 21.49) -> (57.2802, 20.29) centre (58.46, 20.31) ccw
  arc A34 (57.2802, 17.79) -> (58.46, 16.59) centre (58.46, 17.77) ccw
  line L105 (55.16, 17.79) -> (57.2802, 17.79)
  line L106 (55.16, 20.29) -> (57.2802, 20.29)
  arc A35 (55.16, 20.29) -> (55.16, 17.79) centre (55.16, 19.04) ccw
  line L107 (61, 11.51) -> (58.46, 11.51)
  line L108 (61, 16.41) -> (61, 11.51)
  line L109 (61, 16.41) -> (58.46, 16.41)
  arc A36 (58.46, 16.41) -> (57.2802, 15.21) centre (58.46, 15.23) ccw
  arc A37 (57.2802, 12.71) -> (58.46, 11.51) centre (58.46, 12.69) ccw
  line L110 (55.16, 12.71) -> (57.2802, 12.71)
  line L111 (55.16, 15.21) -> (57.2802, 15.21)
  arc A38 (55.16, 15.21) -> (55.16, 12.71) centre (55.16, 13.96) ccw
  line L112 (61, 6.43) -> (58.46, 6.43)
  line L113 (61, 11.33) -> (61, 6.43)
  line L114 (61, 11.33) -> (58.46, 11.33)
  arc A39 (58.46, 11.33) -> (57.2802, 10.13) centre (58.46, 10.15) ccw
  arc A40 (57.2802, 7.63) -> (58.46, 6.43) centre (58.46, 7.61) ccw
  line L115 (55.16, 7.63) -> (57.2802, 7.63)
  line L116 (55.16, 10.13) -> (57.2802, 10.13)
  arc A41 (55.16, 10.13) -> (55.16, 7.63) centre (55.16, 8.88) ccw
  point P0 (0, 0)
  point P1 (61, 21.58)
  dimension "d111" = 4.9
  dimension "d112" = 2.5
  dimension "d115" = 5.08
  constraints: 40 end point, 24 point on circle, 12 centre point, 3 coincident, 3 horizontal, 3 tangent, 2 midpoint, 2 parallel, 2 point on line, 1 collinear, 1 equal radius, 1 perpendicular, 1 vertical, 57 other
  measures "d111" distance between parallel lines of L97 L96
  measures "d112" distance between parallel lines of L100 L99
  measures "d115" distance of L97.start L102.start
extrude "Extrusion13" cut sketch "Sketch13" against normal blind 0.01 contours L113 A0 | A0 L11 L112 A40 L115 A41 L116 A39 L114 L1 A1 L0 | A1 L113 | L107 A37 L110 A38 L111 A36 L109 L3 A3 L2 A2 L1 | A2 L108 | A3 L108 | L102 A34 L105 A35 L106 A33 L104 L5 A5 L4 A4 L3 | L7 A7 L6 A6 L5 L97 A31 L100 A32 L99 A30 L96 | A4 L103 | A5 L103
sketch "Sketch14" plane through (0, 0, 0) normal (0, 0, -1) x (-1, 0, 0)
  arc A0 (-61, 12.29) -> (-61, 13.09) centre (-61, 12.69) ccw projected
  line L0 (-61, 14.83) -> (-61, 13.09) projected
  arc A1 (-61, 14.83) -> (-61, 15.63) centre (-61, 15.23) ccw projected
  line L1 (-61, 16.41) -> (-61, 15.63) projected
  line L2 (-58.46, 16.41) -> (-61, 16.41) projected
  arc A2 (-57.2802, 15.21) -> (-58.46, 16.41) centre (-58.46, 15.23) ccw projected
  line L3 (-55.16, 15.21) -> (-57.2802, 15.21) projected
  arc A3 (-55.16, 12.71) -> (-55.16, 15.21) centre (-55.16, 13.96) ccw projected
  line L4 (-57.2802, 12.71) -> (-55.16, 12.71) projected
  arc A4 (-58.46, 11.51) -> (-57.2802, 12.71) centre (-58.46, 12.69) ccw projected
  line L5 (-61, 11.51) -> (-58.46, 11.51) projected
  line L6 (-61, 12.29) -> (-61, 11.51) projected
  circle A5 centre (-55.16, 13.96) radius 0.4 projected
  circle A6 centre (-58.46, 15.23) radius 0.4 projected
  circle A7 centre (-58.46, 12.69) radius 0.4 projected
  arc A8 (-61, 7.21) -> (-61, 8.01) centre (-61, 7.61) ccw projected
  line L7 (-61, 9.75) -> (-61, 8.01) projected
  arc A9 (-61, 9.75) -> (-61, 10.55) centre (-61, 10.15) ccw projected
  line L8 (-61, 11.33) -> (-61, 10.55) projected
  line L9 (-58.46, 11.33) -> (-61, 11.33) projected
  arc A10 (-57.2802, 10.13) -> (-58.46, 11.33) centre (-58.46, 10.15) ccw projected
  line L10 (-55.16, 10.13) -> (-57.2802, 10.13) projected
  arc A11 (-55.16, 7.63) -> (-55.16, 10.13) centre (-55.16, 8.88) ccw projected
  line L11 (-57.2802, 7.63) -> (-55.16, 7.63) projected
  arc A12 (-58.46, 6.43) -> (-57.2802, 7.63) centre (-58.46, 7.61) ccw projected
  line L12 (-61, 6.43) -> (-58.46, 6.43) projected
  line L13 (-61, 7.21) -> (-61, 6.43) projected
  circle A13 centre (-58.46, 10.15) radius 0.4 projected
  circle A14 centre (-58.46, 7.61) radius 0.4 projected
  circle A15 centre (-55.16, 8.88) radius 0.4 projected
  arc A16 (-61, 17.37) -> (-61, 18.17) centre (-61, 17.77) ccw projected
  line L14 (-61, 19.91) -> (-61, 18.17) projected
  arc A17 (-61, 19.91) -> (-61, 20.71) centre (-61, 20.31) ccw projected
  line L15 (-61, 21.49) -> (-61, 20.71) projected
  line L16 (-58.46, 21.49) -> (-61, 21.49) projected
  arc A18 (-57.2802, 20.29) -> (-58.46, 21.49) centre (-58.46, 20.31) ccw projected
  line L17 (-55.16, 20.29) -> (-57.2802, 20.29) projected
  arc A19 (-55.16, 17.79) -> (-55.16, 20.29) centre (-55.16, 19.04) ccw projected
  line L18 (-57.2802, 17.79) -> (-55.16, 17.79) projected
  arc A20 (-58.46, 16.59) -> (-57.2802, 17.79) centre (-58.46, 17.77) ccw projected
  line L19 (-61, 16.59) -> (-58.46, 16.59) projected
  line L20 (-61, 17.37) -> (-61, 16.59) projected
  circle A21 centre (-58.46, 20.31) radius 0.4 projected
  circle A22 centre (-58.46, 17.77) radius 0.4 projected
  circle A23 centre (-55.16, 19.04) radius 0.4 projected
  circle A24 centre (-55.16, 24.12) radius 0.4 projected
  circle A25 centre (-58.46, 25.39) radius 0.4 projected
  circle A26 centre (-58.46, 22.85) radius 0.4 projected
  arc A27 (-61, 22.45) -> (-61, 23.25) centre (-61, 22.85) ccw projected
  line L21 (-61, 24.99) -> (-61, 23.25) projected
  arc A28 (-61, 24.99) -> (-61, 25.79) centre (-61, 25.39) ccw projected
  line L22 (-61, 26.57) -> (-61, 25.79) projected
  line L23 (-58.46, 26.57) -> (-61, 26.57) projected
  arc A29 (-57.2802, 25.37) -> (-58.46, 26.57) centre (-58.46, 25.39) ccw projected
  line L24 (-55.16, 25.37) -> (-57.2802, 25.37) projected
  arc A30 (-55.16, 22.87) -> (-55.16, 25.37) centre (-55.16, 24.12) ccw projected
  line L25 (-57.2802, 22.87) -> (-55.16, 22.87) projected
  arc A31 (-58.46, 21.67) -> (-57.2802, 22.87) centre (-58.46, 22.85) ccw projected
  line L26 (-61, 21.67) -> (-58.46, 21.67) projected
  line L27 (-61, 22.45) -> (-61, 21.67) projected
  point P0 (0, 0)
extrude "Extrusion14" cut sketch "Sketch14" against normal blind 0.01
body "Solid1"
